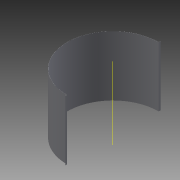
# Autodesk Inventor part: New Band Design
Saved by Autodesk Inventor 2015 (Build 190159000, 159)
## iProperties
Created: 2014-06-23
Part Number: New Band Design
Material: Generic
Document SubType Name: Modeling
Designer: Aki
Density: 1 g/cm^3
Appearance: Default
Author: Aki
Autodesk Inventor part; units mm, degrees
ref_plane "YZ Plane" through (0, 0, 0) normal (1, 0, 0) x (0, 1, 0)
ref_plane "XZ Plane" through (0, 0, 0) normal (0, 1, 0) x (-1, 0, 0)
ref_plane "XY Plane" through (0, 0, 0) normal (0, 0, 1) x (1, 0, 0)
sketch "Sketch1" plane through (0, 0, 0) normal (0, 1, 0) x (-1, 0, 0)
  arc A0 (0, -401) -> (0, 401) centre (0, 0) ccw
  line L0 (0, 0) -> (0, 401) construction
  line L1 (0, 0) -> (0, -401) construction
  arc A1 (0, -400) -> (0, 400) centre (0, 0) ccw
  line L2 (0, 0) -> (0, 400) construction
  line L3 (0, 0) -> (0, -400) construction
  line L4 (0, 401) -> (0, 400)
  line L5 (0, -401) -> (0, -400)
  dimension "d0" = 401
  dimension "d1" = 180
  dimension "d2" = 400
  dimension "d3" = 180
  constraints: 12 end point, 4 point on circle, 2 centre point, 2 coincident, 1 collinear, 1 point on line
  measures "d0" radius of A0
  measures "d1" angle of L0 L1
  measures "d2" radius of A1
  measures "d3" angle of L2 L3
extrude "Extrusion1" add sketch "Sketch1" along normal blind 523.3
sketch "Sketch2" plane through (0, 0, 0) normal (0, 1, 0) x (-1, 0, 0)
  line L0 (0, 401) -> (1, 401)
  line L1 (1, 401) -> (1, 416)
  line L2 (1, 416) -> (0, 416)
  line L3 (0, 416) -> (0, 401)
  point P0 (0, 0)
  dimension "d6" = 1
  dimension "d7" = 15
  constraints: 8 end point, 2 parallel, 1 horizontal, 1 perpendicular
  measures "d6" distance of L2.end L1.end
  measures "d7" distance of L1.end L0.end
extrude "Extrusion2" add sketch "Sketch2" along normal blind 523.3
sketch "Sketch3" plane through (0, 0, 0) normal (0, 1, 0) x (-1, 0, 0)
  line L0 (0, -401) -> (1, -401)
  line L1 (1, -401) -> (1, -416)
  line L2 (1, -416) -> (0, -416)
  line L3 (0, -416) -> (0, -401)
  point P0 (0, 0)
  dimension "d12" = 1
  dimension "d13" = 15
  constraints: 8 end point, 2 parallel, 1 horizontal, 1 perpendicular
  measures "d12" distance of L1.end L2.end
  measures "d13" distance of L0.end L1.end
extrude "Extrusion3" add sketch "Sketch3" along normal blind 523.3
body "Solid1"
